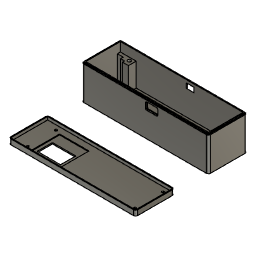
3d_case_sim7000g (Autodesk Fusion 360 design; units mm, degrees)
Autodesk Fusion 360 part; units mm, degrees
sketch "Boceto1" plane through (0, 0, 0) normal (0, 0, 1) x (1, 0, 0)
  line L0 (0, 0) -> (125, 0)
  line L1 (125, 0) -> (125, -40)
  line L2 (125, -40) -> (0, -40)
  line L3 (0, -40) -> (0, 0)
  line L4 (1, -1) -> (124, -1)
  line L5 (124, -1) -> (124, -39)
  line L6 (124, -39) -> (1, -39)
  line L7 (1, -39) -> (1, -1)
  line L8 (2, -2) -> (123, -2)
  line L9 (123, -2) -> (123, -38)
  line L10 (123, -38) -> (2, -38)
  line L11 (2, -38) -> (2, -2)
  line L12 (2, -2) -> (12.5, -2)
  line L13 (12.5, -2) -> (12.5, -6.8)
  line L14 (12.5, -6.8) -> (2, -6.8)
  line L15 (2, -6.8) -> (2, -2)
  line L16 (2, -38) -> (12.5, -38)
  line L17 (12.5, -38) -> (12.5, -33.2)
  line L18 (12.5, -33.2) -> (2, -33.2)
  line L19 (2, -33.2) -> (2, -38)
  line L20 (123, -2) -> (116, -2)
  line L21 (116, -2) -> (116, -10.4)
  line L22 (116, -10.4) -> (123, -10.4)
  line L23 (123, -10.4) -> (123, -2)
  line L24 (123, -38) -> (116, -38)
  line L25 (116, -38) -> (116, -29.6)
  line L26 (116, -29.6) -> (123, -29.6)
  line L27 (123, -29.6) -> (123, -38)
  line L28 (2, -6.8) -> (7.7, -6.8)
  line L29 (7.7, -6.8) -> (7.7, -33.2)
  line L30 (7.7, -33.2) -> (2, -33.2)
  line L31 (2, -33.2) -> (2, -6.8)
  line L32 (7.7, -6.8) -> (9, -6.8)
  line L33 (9, -6.8) -> (9, -9.4)
  line L34 (9, -9.4) -> (7.7, -9.4)
  line L35 (7.7, -9.4) -> (7.7, -6.8)
  line L36 (7.7, -33.2) -> (9, -33.2)
  line L37 (9, -33.2) -> (9, -30.6)
  line L38 (9, -30.6) -> (7.7, -30.6)
  line L39 (7.7, -30.6) -> (7.7, -33.2)
  line L40 (9, -9.4) -> (7.7, -9.4)
  line L41 (7.7, -9.4) -> (7.7, -30.6)
  line L42 (7.7, -30.6) -> (9, -30.6)
  line L43 (9, -30.6) -> (9, -9.4)
  line L44 (11.4716, -4.2311) -> (122.0116, -4.2311)
  line L45 (122.0116, -4.2311) -> (122.0116, -37.1211)
  line L46 (122.0116, -37.1211) -> (11.4716, -37.1211)
  line L47 (11.4716, -37.1211) -> (11.4716, -4.2311)
  line L48 (13.7516, -6.8211, 23) -> (119.3416, -6.8211, 23)
  line L49 (119.3416, -6.8211, 23) -> (119.3416, -34.5311, 23)
  line L50 (119.3416, -34.5311, 23) -> (13.7516, -34.5311, 23)
  line L51 (13.7516, -34.5311, 23) -> (13.7516, -6.8211, 23)
  line L52 (9, -30.6) -> (12.5, -30.6)
  line L53 (12.5, -30.6) -> (12.5, -33.2)
  line L54 (12.5, -33.2) -> (9, -33.2)
  line L55 (9, -33.2) -> (9, -30.6)
  line L56 (12.5, -38) -> (17.5, -38)
  line L57 (17.5, -38) -> (17.5, -30.6)
  line L58 (17.5, -30.6) -> (12.5, -30.6)
  line L59 (12.5, -30.6) -> (12.5, -38)
  line L60 (9, -9.4) -> (12.5, -9.4)
  line L61 (12.5, -9.4) -> (12.5, -6.8)
  line L62 (12.5, -6.8) -> (9, -6.8)
  line L63 (9, -6.8) -> (9, -9.4)
  line L64 (12.5, -9.4) -> (17.5, -9.4)
  line L65 (17.5, -9.4) -> (17.5, -2)
  line L66 (17.5, -2) -> (12.5, -2)
  line L67 (12.5, -2) -> (12.5, -9.4)
  line L68 (125, -40) -> (0, -40)
  line L69 (0, -40) -> (0, 0)
  line L70 (0, 0) -> (125, 0)
  line L71 (125, 0) -> (125, -40)
  line L72 (124, -1) -> (124, -39)
  line L73 (123, -2) -> (123, -38)
  line L74 (1, -1) -> (124, -1)
  line L75 (2, -2) -> (123, -2)
  line L76 (123, -38) -> (2, -38)
  line L77 (124, -39) -> (1, -39)
  line L78 (2, -38) -> (2, -2)
  line L79 (1, -39) -> (1, -1)
  line L80 (119.3416, -34.5311, 23) -> (13.7516, -34.5311, 23)
  line L81 (13.7516, -34.5311, 23) -> (13.7516, -6.8211, 23)
  line L82 (13.7516, -6.8211, 23) -> (119.3416, -6.8211, 23)
  line L83 (119.3416, -6.8211, 23) -> (119.3416, -34.5311, 23)
  line L84 (125.2069, -155.8563) -> (0.2069, -155.8563)
  line L85 (0.2069, -155.8563) -> (0.2069, -115.8563)
  line L86 (0.2069, -115.8563) -> (125.2069, -115.8563)
  line L87 (1.2069, -154.8563) -> (1.2069, -116.8563)
  line L88 (1.2069, -116.8563) -> (124.2069, -116.8563)
  line L89 (124.2069, -154.8563) -> (1.2069, -154.8563)
  line L90 (2.2069, -153.8563) -> (2.2069, -117.8563)
  line L91 (123.2069, -153.8563) -> (2.2069, -153.8563)
  line L92 (125.2069, -115.8563) -> (125.2069, -155.8563)
  line L93 (124.2069, -116.8563) -> (124.2069, -154.8563)
  line L94 (123.2069, -117.8563) -> (123.2069, -153.8563)
  line L95 (2.2069, -117.8563) -> (123.2069, -117.8563)
  line L96 (13.9585, -122.6775) -> (119.5485, -122.6775)
  line L97 (13.9585, -150.3875) -> (13.9585, -122.6775)
  line L98 (119.5485, -150.3875) -> (13.9585, -150.3875)
  line L99 (119.5485, -122.6775) -> (119.5485, -150.3875)
  dimension "d1" = 125
  dimension "d2" = 40
  dimension "d9" = 110.54
  dimension "d10" = 32.89
  dimension "d11" = 105.59
  dimension "d12" = 27.71
  dimension "d15" = 5
  dimension "d16" = 5
  dimension "d41" = 125
  dimension "d42" = 40
  dimension "d43" = 105.59
  dimension "d44" = 27.71
  dimension "d45" = 125
  dimension "d46" = 40
  dimension "d47" = 105.59
  dimension "d48" = 27.71
  constraint horizontal L0
  constraint vertical L1
  constraint horizontal L2
  constraint vertical L3
  constraint coincident L0.start L3.end
  constraint horizontal L4
  constraint vertical L5
  constraint horizontal L6
  constraint vertical L7
  constraint horizontal L8
  constraint vertical L9
  constraint horizontal L10
  constraint vertical L11
  constraint horizontal L12
  constraint vertical L13
  constraint horizontal L14
  constraint vertical L15
  constraint horizontal L16
  constraint vertical L17
  constraint horizontal L18
  constraint vertical L19
  constraint horizontal L20
  constraint vertical L21
  constraint horizontal L22
  constraint vertical L23
  constraint horizontal L24
  constraint vertical L25
  constraint horizontal L26
  constraint vertical L27
  constraint horizontal L28
  constraint vertical L29
  constraint horizontal L30
  constraint vertical L31
  constraint coincident L18 L29.end
  constraint horizontal L32
  constraint vertical L33
  constraint horizontal L34
  constraint vertical L35
  constraint horizontal L36
  constraint vertical L37
  constraint horizontal L38
  constraint vertical L39
  constraint horizontal L40
  constraint vertical L41
  constraint horizontal L42
  constraint vertical L43
  constraint horizontal L44
  constraint vertical L45
  constraint horizontal L46
  constraint vertical L47
  constraint horizontal L52
  constraint vertical L53
  constraint horizontal L54
  constraint vertical L55
  constraint horizontal L56
  constraint vertical L57
  constraint horizontal L58
  constraint vertical L59
  constraint horizontal L60
  constraint vertical L61
  constraint horizontal L62
  constraint vertical L63
  constraint horizontal L64
  constraint vertical L65
  constraint horizontal L66
  constraint vertical L67
  constraint coincident L8 L65.end
  constraint horizontal L70
  constraint vertical L71
  constraint horizontal L68
  constraint vertical L69
  constraint horizontal L74
  constraint vertical L72
  constraint horizontal L77
  constraint vertical L79
  constraint horizontal L75
  constraint vertical L73
  constraint horizontal L76
  constraint vertical L78
  constraint horizontal L86
  constraint horizontal L84
  constraint vertical L85
  constraint vertical L93
  constraint horizontal L89
  constraint vertical L87
  constraint horizontal L95
  constraint vertical L94
  constraint horizontal L91
  constraint vertical L90
  constraint vertical L99
  constraint vertical L92
  constraint horizontal L88
  constraint horizontal L96
  constraint horizontal L98
  constraint vertical L97
  measures "d1" distance of L0.start L0.end
  measures "d2" distance of L0.start L2.end
  measures "d9" distance of L44.start L44.end
  measures "d10" distance of L44.start L46.end
  measures "d15" distance of L16.end L56.end
  measures "d16" distance of L60.end L64.end
  measures "d41" distance of L0.start L0.end
  measures "d42" distance of L0.start L2.end
  measures "d45" distance of L85.end L86.end
  measures "d46" distance of L85.end L84.end
  measures "d47" distance of L96.end L96.start
  measures "d48" distance of L96.start L97.start
extrude "Extruir1" add sketch "Boceto1" against normal blind 2 contours L0 L1 L2 L3 L68 L69 L70 L71 | L4 L5 L6 L7 L72 L74 L77 L79 | L8 L11 L12 L13 L14 L15 L28 L32 L44 L47 L62 L67 L75 L78 | L8 L13 L44 L65 L66 L67 L75 | L11 L14 L18 L28 L29 L30 L31 L35 L39 L41 L78 | L8 L21 L44 L65 L75 | L13 L44 L61 L64 L65 L67 | L13 L14 L44 L47 L62 L67 | L10 L11 L16 L17 L18 L19 L30 L36 L46 L47 L54 L59 L76 L78 | L14 L29 L32 L33 L34 L35 L40 L63 | L8 L9 L20 L21 L22 L23 L44 L45 L73 L75 | L21 L22 L25 L26 L44 L45 L46 L47 L52 L57 L58 L60 L64 L65 | L14 L47 L60 L61 L62 L67 | L18 L29 L36 L37 L38 L39 L42 L55 | L14 L33 L47 L60 L62 L63 | L29 L34 L38 L40 L41 L42 L43 | L21 L22 L44 L45 | L10 L17 L46 L56 L57 L59 L76 | L18 L37 L47 L52 L54 L55 | L43 L47 L52 L60 | L9 L22 L26 L45 L73 | L10 L25 L46 L57 L76 | L17 L18 L46 L47 L54 L59 | L17 L46 L53 L57 L58 L59 | L18 L47 L52 L53 L54 L59 | L9 L10 L24 L25 L26 L27 L45 L46 L73 L76 | L25 L26 L45 L46 makes body 1
extrude "Extruir2" add sketch "Boceto1" along normal blind 32 contours L4 L5 L6 L7 L72 L74 L77 L79 bodies 1
extrude "Extruir3" add sketch "Boceto1" along normal blind 30 contours L0 L1 L2 L3 L68 L69 L70 L71 bodies 1
sketch "Boceto3" plane through (0, -40, 0) normal (0, -1, 0) x (1, 0, 0)
  line L0 (0, 30) -> (0, -2)
  line L1 (0, -2) -> (125, -2)
  line L2 (125, -2) -> (125, 30)
  line L3 (125, 30) -> (0, 30)
  line L4 (63.5, 29) -> (74.5, 29)
  line L5 (74.5, 29) -> (74.5, 23)
  line L6 (74.5, 23) -> (63.5, 23)
  line L7 (63.5, 23) -> (63.5, 29)
  dimension "d23" = 50.5
  dimension "d24" = 63.5
  dimension "d25" = 23
  dimension "d26" = 6
  constraint horizontal L4
  constraint vertical L5
  constraint horizontal L6
  constraint vertical L7
  measures "d23" horizontal distance of L1.end L5.end
  measures "d24" horizontal distance of L0.end L6.end
  measures "d25" vertical distance of origin L6.end
  measures "d26" distance of L4.start L6.end
extrude "Extruir4" cut sketch "Boceto3" against normal blind 3 contours L4 L5 L6 L7 bodies 1
fillet "Empalme1" radius 0.6 4 faces at (63.5, -39.3333, 25) (70.8333, -39.3333, 23) (74.5, -39.3333, 27) (67.1667, -39.3333, 29) on bodies 1
sketch "Boceto4" plane through (0, -40, 0) normal (0, -1, 0) x (1, 0, 0)
  line L0 (0, 30) -> (0, -2)
  line L1 (0, -2) -> (125, -2)
  line L2 (125, -2) -> (125, 30)
  line L3 (125, 30) -> (0, 30)
  arc A0 (64.1, 29.6) -> (62.9, 28.4) centre (64.1, 28.4) ccw
  line L4 (64.1, 29.6) -> (73.9, 29.6)
  arc A1 (75.1, 28.4) -> (73.9, 29.6) centre (73.9, 28.4) ccw
  line L5 (75.1, 28.4) -> (75.1, 23.6)
  arc A2 (73.9, 22.4) -> (75.1, 23.6) centre (73.9, 23.6) ccw
  line L6 (73.9, 22.4) -> (64.1, 22.4)
  arc A3 (62.9, 23.6) -> (64.1, 22.4) centre (64.1, 23.6) ccw
  line L7 (62.9, 23.6) -> (62.9, 28.4)
sketch "Boceto5" plane through (0, 0, 0) normal (0, 1, 0) x (-1, 0, 0)
  line L0 (-125, 30) -> (-125, -2)
  line L1 (-125, -2) -> (0, -2)
  line L2 (0, -2) -> (0, 30)
  line L3 (0, 30) -> (-125, 30)
  line L4 (-74, 28.7) -> (-67.5, 28.7)
  line L5 (-67.5, 28.7) -> (-67.5, 25)
  line L6 (-67.5, 25) -> (-74, 25)
  line L7 (-74, 25) -> (-74, 28.7)
  line L8 (0, 0) -> (-125, 0)
  dimension "d31" = 51
  dimension "d32" = 67.5
  dimension "d33" = 25
  dimension "d34" = 3.7
  constraint horizontal L4
  constraint vertical L5
  constraint horizontal L6
  constraint vertical L7
  measures "d31" horizontal distance of L0.end L6.end
  measures "d32" horizontal distance of L1.end L5.end
  measures "d33" distance of L6.end L8
  measures "d34" distance of L4.start L6.end
extrude "Extruir5" add 1 faces at (42, -0.3333, 30) along direction (0, 0, 1) blind 1 on bodies 1 bodies 1
extrude "Extruir6" cut sketch "Boceto5" against normal blind 3 contours L4 L5 L6 L7 bodies 1
fillet "Empalme2" radius 0.5 4 faces at (69.6667, -0.6667, 25) (67.5, -0.6667, 27.4667) (71.8333, -0.6667, 28.7) (74, -0.6667, 26.2333) on bodies 1
extrude "Extruir7" add sketch "Boceto1" along normal blind 23 contours L8 L11 L12 L13 L14 L15 L28 L32 L44 L47 L62 L67 L75 L78 | L8 L13 L44 L65 L66 L67 L75 | L13 L44 L61 L64 L65 L67 | L13 L14 L44 L47 L62 L67 | L10 L11 L16 L17 L18 L19 L30 L36 L46 L47 L54 L59 L76 L78 | L14 L29 L32 L33 L34 L35 L40 L63 | L8 L9 L20 L21 L22 L23 L44 L45 L73 L75 | L14 L47 L60 L61 L62 L67 | L18 L29 L36 L37 L38 L39 L42 L55 | L14 L33 L47 L60 L62 L63 | L21 L22 L44 L45 | L10 L17 L46 L56 L57 L59 L76 | L18 L37 L47 L52 L54 L55 | L17 L18 L46 L47 L54 L59 | L17 L46 L53 L57 L58 L59 | L18 L47 L52 L53 L54 L59 | L9 L10 L24 L25 L26 L27 L45 L46 L73 L76 | L25 L26 L45 L46 bodies 1
extrude "Extruir8" add sketch "Boceto1" along normal blind 2 contours L29 L34 L38 L40 L41 L42 L43 bodies 1
extrude "Extruir9" add sketch "Boceto1" against normal blind 2 separate body contours L84 L85 L86 L92 | L87 L88 L89 L93 | L90 L91 L94 L95 | L96 L97 L98 L99 makes body 2
sketch "Boceto6" plane through (0, 0, 0) normal (0, 0, 1) x (1, 0, 0)
  line L0 (44.9828, -145.874) -> (21.9828, -145.874)
  line L1 (21.9828, -145.874) -> (21.9828, -121.874)
  line L2 (21.9828, -121.874) -> (44.9828, -121.874)
  line L3 (44.9828, -121.874) -> (44.9828, -145.874)
  line L4 (44.9841, -138.874) -> (21.9841, -138.874)
  line L5 (21.9841, -138.874) -> (21.9841, -123.874)
  line L6 (21.9841, -123.874) -> (44.896, -123.874)
  line L7 (44.896, -123.874) -> (44.9841, -138.874)
  dimension "d55" = 23
  dimension "d56" = 24
  dimension "d58" = 15
  dimension "d59" = 23
  measures "d55" distance of L0.start L0.end
  measures "d56" distance of L0.start L2.end
  measures "d58" distance of L4.end L5.end
  measures "d59" distance of L4.start L4.end
hole "Agujero1" at (13.7516, -6.8211, 23) at (13.7516, -34.5311, 23) at (119.3416, -6.8211, 23) at (119.3416, -34.5311, 23) direction (0, 0, -1) diameter 3.2 depth 9 tip angle 180 bodies 1
sketch "Boceto7" plane through (0, 0, -2) normal (0, 0, -1) x (1, 0, 0)
  line L0 (0.2069, 115.8563) -> (125.2069, 115.8563)
  line L1 (125.2069, 115.8563) -> (125.2069, 155.8563)
  line L2 (125.2069, 155.8563) -> (0.2069, 155.8563)
  line L3 (0.2069, 155.8563) -> (0.2069, 115.8563)
  line L4 (0.2069, 155.8563) -> (125.2069, 155.8563)
  line L5 (125.2069, 155.8563) -> (125.2069, 115.8563)
  line L6 (125.2069, 115.8563) -> (0.2069, 115.8563)
  line L7 (0.2069, 115.8563) -> (0.2069, 155.8563)
  line L8 (1.2069, 154.8563) -> (124.2069, 154.8563)
  line L9 (124.2069, 154.8563) -> (124.2069, 116.8563)
  line L10 (124.2069, 116.8563) -> (1.2069, 116.8563)
  line L11 (1.2069, 116.8563) -> (1.2069, 154.8563)
  point P0 (125.2069, 115.8563)
  point P1 (125.2069, 155.8563)
  dimension "d63" = 1
  dimension "d64" = 1
  dimension "d66" = 1
  dimension "d67" = 1
  constraint horizontal L4
  constraint vertical L5
  constraint horizontal L6
  constraint vertical L7
  constraint coincident P0 L0.end
  constraint coincident L2.end L3.start
  constraint horizontal L8
  constraint vertical L9
  constraint horizontal L10
  constraint vertical L11
  measures "d63" horizontal distance of L2.end L8.start
  measures "d64" vertical distance of L0.start L10.end
  measures "d66" vertical distance of L2.end L8.start
  measures "d67" horizontal distance of L8.end P1
extrude "Extruir10" add sketch "Boceto7" along normal blind 3 bodies 2
sketch "Boceto8" plane through (0, 0, 0) normal (0, 0, 1) x (1, 0, 0)
  circle A0 through (15.9556, -150.381, 5) (12.9556, -148.649, 5) (12.9556, -152.1131, 5)
  circle A1 through (15.1056, -150.381, 5) (13.3806, -149.3851, 5) (13.3806, -151.3769, 5)
  circle A2 through (15.9556, -122.6758, 5) (12.9556, -120.9438, 5) (12.9556, -124.4079, 5)
  circle A3 through (15.1056, -122.6758, 5) (13.3806, -121.6799, 5) (13.3806, -123.6718, 5)
  circle A4 through (121.544, -122.6758, 5) (118.544, -120.9438, 5) (118.544, -124.4079, 5)
  circle A5 through (120.694, -122.6758, 5) (118.969, -121.6799, 5) (118.969, -123.6718, 5)
  circle A6 through (121.5337, -150.3912, 5) (118.5337, -148.6592, 5) (118.5337, -152.1233, 5)
  circle A7 through (120.6837, -150.3912, 5) (118.9587, -149.3953, 5) (118.9587, -151.3872, 5)
  dimension "d70" = 4
  dimension "d71" = 2.3
  dimension "d72" = 4
  dimension "d73" = 2.3
  dimension "d74" = 4
  dimension "d75" = 2.3
  dimension "d76" = 4
  dimension "d77" = 2.3
extrude "Extruir11" cut sketch "Boceto6" against normal blind 2 contours L1 L4 L5 L6 L7 bodies 2
fillet "Empalme3" radius 2 1 edges at (125, -40, 14.5) on bodies 1
fillet "Empalme4" radius 2 1 edges at (125, 0, 14.5) on bodies 1
fillet "Empalme5" radius 2 1 edges at (0, -40, 14.5) on bodies 1
fillet "Empalme6" radius 2 1 edges at (0, 0, 14.5) on bodies 1
fillet "Empalme7" radius 2 1 edges at (0.2069, -155.8563, -2.5) on bodies 2
fillet "Empalme8" radius 2 1 edges at (0.2069, -115.8563, -2.5) on bodies 2
fillet "Empalme9" radius 2 1 edges at (125.2069, -155.8563, -2.5) on bodies 2
fillet "Empalme10" radius 2 1 edges at (125.2069, -115.8563, -2.5) on bodies 2
extrude "Extruir12" cut sketch "Boceto8" against normal blind 0.5 contours A0 | A1 | A2 | A3 | A4 | A5 | A6 | A7 in plane through (0, 0, 5) normal (0, 0, 1) bodies 2
hole "Agujero2" at (13.9585, -150.3875, 0) at (13.9585, -122.6775, 0) at (119.5485, -150.3875, 0) at (119.5485, -122.6775, 0) direction (0, 0, -1) diameter 2.05 depth 2 tip angle 180 bodies 2
extrude "Extruir13" add 1 faces at (67.1667, -2, 8.1667) along direction (0, -1, 0) blind 1.8 on bodies 1 bodies 1
extrude "Extruir14" cut 1 faces at (42, -1, 31.6667) along direction (0, -1, 0) blind 1.8 on bodies 1 bodies 1
extrude "Extruir15" cut 1 faces at (23.675, 0, 18.0925) along direction (0, -1, 0) blind 1.8 on bodies 1 bodies 1
extrude "Extruir16" cut 1 faces at (2, -0.6, 9) along direction (-1, 0, 0) blind 2 on bodies 1 bodies 1
extrude "Extruir17" cut 1 faces at (123, -0.6, 20) along direction (1, 0, 0) blind 2 on bodies 1 bodies 1
extrude "Extruir18" cut sketch "Boceto5" against normal blind 1.8 contours L0 L2 L3 L8 | L4 L5 L6 L7 bodies 1
delete_face "SuprimirCaras1" 1 faces at (67.0496, -1.9995, 25.2694) on bodies 1
delete_face "SuprimirCaras2" 1 faces at (71.431, -1.911, 24.7848) on bodies 1
delete_face "SuprimirCaras3" 1 faces at (67.3752, -1.8305, 27.042) on bodies 1
delete_face "SuprimirCaras4" 1 faces at (68.4805, -1.9999, 29.0662) on bodies 1
delete_face "SuprimirCaras5" 1 faces at (73.8608, -1.9999, 26.445) on bodies 1
delete_face "SuprimirCaras6" 1 faces at (74.1161, -1.8203, 26.1333) on bodies 1
delete_face "SuprimirCaras7" 1 faces at (72.555, -1.9999, 28.5608) on bodies 1
delete_face "SuprimirCaras8" 1 faces at (67.8107, -3.1333, 24.5181) on bodies 1
delete_face "SuprimirCaras9" 1 faces at (73.6893, -3.1333, 24.5181) on bodies 1
delete_face "SuprimirCaras10" 1 faces at (74.3004, -3.1333, 28.7995) on bodies 1
delete_face "SuprimirCaras11" 1 faces at (67.1996, -3.1333, 28.7995) on bodies 1
fillet "Empalme11" radius 3.5 1 edges at (70.75, -1.8, 24.5) on bodies 1
fillet "Empalme12" radius 1 1 edges at (74.5, -1.8, 25.0689) on bodies 1
fillet "Empalme13" radius 1 1 edges at (67, -1.8, 25.0689) on bodies 1
fillet "Empalme14" radius 2 1 edges at (124.99, -1.8, 14.5) on bodies 1
fillet "Empalme15" radius 2 1 edges at (0.01, -1.8, 14.5) on bodies 1
extrude "Extruir19" add 1 faces at (83.2069, -116.8563, -3) along direction (0, -1, 0) blind 1.8 on bodies 2 bodies 2
extrude "Extruir20" cut 1 faces at (82.8735, -115.8563, -3.3333) along direction (0, -1, 0) blind 1.8 on bodies 2 bodies 2
extrude "Extruir21" cut 1 faces at (2.2069, -117.0563, -1.6667) along direction (-1, 0, 0) blind 2 on bodies 2 bodies 2
extrude "Extruir22" cut 1 faces at (123.2069, -116.4563, -3.3333) along direction (1, 0, 0) blind 2 on bodies 2 bodies 2
fillet "Empalme16" radius 2 1 edges at (125.1969, -117.6563, -2.5) on bodies 2
fillet "Empalme17" radius 2 1 edges at (0.2169, -117.6563, -2.5) on bodies 2
move_body "Desplazar1" bodies 1 to x (1, 0, 0) y (0, 1, 0) z (0, 0, 1) at (0, 0, 2)
move_body "Desplazar2" bodies 2 to x (1, 0, 0) y (0, 1, 0) z (0, 0, 1) at (0, 0, 5)
sketch "Boceto9" plane through (0, -9.4, 0) normal (0, -1, 0) x (1, 0, 0)
  line L0 (7.7, 4) -> (9, 4)
  line L1 (9, 4) -> (9, 2)
  line L2 (9, 2) -> (17.5, 2)
  line L3 (17.5, 2) -> (17.5, 25)
  line L4 (17.5, 25) -> (7.7, 25)
  line L5 (7.7, 25) -> (7.7, 4)
  line L6 (17.5, 25) -> (11.5, 25)
  line L7 (11.5, 25) -> (11.5, 2)
  line L8 (11.5, 2) -> (17.5, 2)
  line L9 (17.5, 2) -> (17.5, 25)
  dimension "d135" = 6
  constraint horizontal L6
  constraint vertical L7
  constraint horizontal L8
  constraint vertical L9
  constraint coincident L3.end L4.start
  measures "d135" distance of L3.end L6.end
extrude "Extruir23" add sketch "Boceto9" along normal blind 2 contours L2 L3 L4 L6 L7 L8 L9 bodies 1
hole "Agujero3" at (13.9556, -150.381, 5) direction (0, 0, -1) diameter 2.3 depth 2 tip angle 180 bodies 2
hole "Agujero4" at (119.5337, -150.3912, 5) direction (0, 0, -1) diameter 2.3 depth 2 tip angle 180 bodies 2
hole "Agujero5" at (119.544, -122.6758, 5) direction (0, 0, -1) diameter 2.3 depth 2 tip angle 180 bodies 2
hole "Agujero6" at (13.9556, -122.6758, 5) direction (0, 0, -1) diameter 2.3 depth 2 tip angle 180 bodies 2
move_body "Desplazar3" bodies 2 to x (1, 0, 0) y (0, -1, 0) z (0, 0, -1) at (0, -311.7126, 0)
move_body "Desplazar4" bodies 2 to x (1, 0, 0) y (0, 1, 0) z (0, 0, 1) at (0, 0, 5)
move_body "Desplazar5" bodies 2 to x (1, 0, 0) y (0, 1, 0) z (0, 0, 1) at (0, 82, 0)
sketch "Boceto10" plane through (0, 0, 0) normal (0, 0, -1) x (1, 0, 0)
  circle A0 centre (13.9556, 107.0368) radius 1.15
  circle A1 centre (119.544, 107.0368) radius 1.15
  circle A2 centre (119.5337, 79.3214) radius 1.15
  circle A3 centre (13.9556, 79.3316) radius 1.15
  arc A4 (2.2069, 112.0563) -> (0.2069, 110.0563) centre (2.2069, 110.0563) ccw
  line L0 (0.2069, 110.0563) -> (0.2069, 75.8563)
  arc A5 (0.2069, 75.8563) -> (2.2069, 73.8563) centre (2.2069, 75.8563) ccw
  line L1 (2.2069, 73.8563) -> (123.2069, 73.8563)
  arc A6 (123.2069, 73.8563) -> (125.2069, 75.8563) centre (123.2069, 75.8563) ccw
  line L2 (125.2069, 75.8563) -> (125.2069, 110.0563)
  arc A7 (125.2069, 110.0563) -> (123.2069, 112.0563) centre (123.2069, 110.0563) ccw
  line L3 (123.2069, 112.0563) -> (2.2069, 112.0563)
  line L4 (21.9841, 90.8386) -> (21.9841, 105.8386)
  line L5 (21.9841, 105.8386) -> (44.896, 105.8386)
  line L6 (44.896, 105.8386) -> (44.9828, 91.0584)
  line L7 (44.9828, 91.0584) -> (44.9828, 90.8386)
  line L8 (44.9828, 90.8386) -> (21.9841, 90.8386)
  circle A8 centre (13.9556, 107.0368) radius 2
  circle A9 centre (13.9556, 79.3316) radius 2
  circle A10 centre (119.5337, 79.3214) radius 2
  circle A11 centre (119.544, 107.0368) radius 2
  dimension "d150" = 4
  dimension "d151" = 4
  dimension "d152" = 4
  dimension "d153" = 4
  constraint concentric A0 A8
  constraint concentric A3 A9
  constraint concentric A2 A10
  constraint concentric A1 A11
  measures "d150" diameter of A8
  measures "d151" diameter of A9
  measures "d152" diameter of A10
  measures "d153" diameter of A11
extrude "Extruir24" cut sketch "Boceto10" against normal blind 1 contours A8 | A9 | A10 | A11 bodies 2
hole "Agujero7" at (13.9556, -107.0368, 1) direction (0, 0, 1) diameter 2.4 depth 2 tip angle 180 bodies 2
hole "Agujero8" at (13.9556, -79.3316, 1) direction (0, 0, 1) diameter 2.4 depth 2 tip angle 180 bodies 2
hole "Agujero9" at (119.5337, -79.3214, 1) direction (0, 0, 1) diameter 2.4 depth 2 tip angle 180 bodies 2
hole "Agujero10" at (119.544, -107.0368, 1) direction (0, 0, 1) diameter 2.4 depth 2 tip angle 180 bodies 2
extrude "Extruir25" cut 1 faces at (42.2069, -74.8563, 3) along direction (0, 1, 0) blind 0.3 on bodies 2 bodies 2
extrude "Extruir26" cut 1 faces at (124.2069, -86.723, 3) along direction (1, 0, 0) blind 0.3 on bodies 2 bodies 2
extrude "Extruir27" cut 1 faces at (1.2069, -86.723, 4) along direction (-1, 0, 0) blind 0.3 on bodies 2 bodies 2
extrude "Extruir28" cut 1 faces at (42.1069, -111.0563, 4) along direction (0, -1, 0) blind 0.3 on bodies 2 bodies 2
sketch "Boceto11" plane through (0, 0, 2) normal (0, 0, 1) x (-1, 0, 0)
  circle A0 centre (-119.544, 107.0368) radius 1.2
  circle A1 centre (-119.5337, 79.3214) radius 1.2
  circle A2 centre (-13.9556, 79.3316) radius 1.2
  circle A3 centre (-13.9556, 107.0368) radius 1.2
  line L0 (-124.5069, 111.3563) -> (-124.5069, 74.5563)
  line L1 (-124.5069, 74.5563) -> (-0.9069, 74.5563)
  line L2 (-0.9069, 74.5563) -> (-0.9069, 111.3563)
  line L3 (-0.9069, 111.3563) -> (-124.5069, 111.3563)
  line L4 (-21.9841, 105.8386) -> (-21.9841, 90.8386)
  line L5 (-21.9841, 90.8386) -> (-44.9828, 90.8386)
  line L6 (-44.9828, 90.8386) -> (-44.9828, 91.0584)
  line L7 (-44.9828, 91.0584) -> (-44.896, 105.8386)
  line L8 (-44.896, 105.8386) -> (-21.9841, 105.8386)
  line L9 (-47.9828, 107.8386) -> (-18.9841, 107.8386)
  line L10 (-18.9841, 107.8386) -> (-18.9841, 85.8386)
  line L11 (-18.9841, 85.8386) -> (-47.9828, 85.8386)
  line L12 (-47.9828, 85.8386) -> (-47.9828, 107.8386)
  dimension "d176" = 3
  dimension "d177" = 3
  dimension "d178" = 2
  dimension "d179" = 5
  constraint horizontal L9
  constraint vertical L10
  constraint horizontal L11
  constraint vertical L12
  measures "d176" horizontal distance of L5.end L11.end
  measures "d177" horizontal distance of L4.end L10.end
  measures "d178" vertical distance of L7.end L9.start
  measures "d179" vertical distance of L4.end L10.end
extrude "Extruir29" cut sketch "Boceto11" against normal blind 0.8 contours L9 L10 L11 L12 bodies 2
extrude "Extruir30" add 1 faces at (0.9069, -86.823, 4) along direction (1, 0, 0) blind 0.2 on bodies 2 bodies 2
extrude "Extruir31" add 1 faces at (83.3735, -74.5563, 3) along direction (0, -1, 0) blind 0.2 on bodies 2 bodies 2
extrude "Extruir32" add 1 faces at (42.2402, -111.3563, 3) along direction (0, 1, 0) blind 0.2 on bodies 2 bodies 2
extrude "Extruir33" add 1 faces at (124.5069, -86.8896, 3) along direction (-1, 0, 0) blind 0.2 on bodies 2 bodies 2
extrude "Extruir34" cut 1 faces at (28.6503, -107.8386, 1.4667) along direction (0, -1, 0) blind 2.5 on bodies 2 bodies 2
extrude "Extruir35" cut 1 faces at (38.3166, -85.8386, 1.4667) along direction (0, 1, 0) blind 4 on bodies 2 bodies 2
extrude "Extruir36" cut 1 faces at (38.3166, -81.8386, 1.4667) along direction (0, 1, 0) blind 1 on bodies 2 bodies 2
